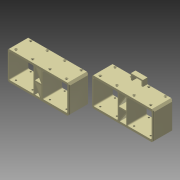
# Autodesk Inventor part: Part6
Saved by Autodesk Inventor 2015 (Build 190159000, 159)
## iProperties
Created: 2015-03-12
Part Number: Part6
Material: Nylon 6/6
Document SubType Name: Modeling
Designer: Vladimir
Density: 1.13 g/cm^3
Appearance: Nylon 6
Author: Vladimir
Autodesk Inventor part; units mm, degrees
ref_plane "YZ Plane" through (0, 0, 0) normal (1, 0, 0) x (0, 1, 0)
ref_plane "XZ Plane" through (0, 0, 0) normal (0, 1, 0) x (-1, 0, 0)
ref_plane "XY Plane" through (0, 0, 0) normal (0, 0, 1) x (1, 0, 0)
sketch "0.2mm tolerance" plane through (0, 0, 0) normal (0, 0, 1) x (1, 0, 0)
  line L0 (-41.2, -0.2479) -> (-41.2, 26.7521)
  line L1 (-13.4, -0.0479) -> (-38, -0.0479)
  line L2 (-39, 0.9521) -> (-39, 25.5521)
  line L3 (-38, 26.5521) -> (-13.4, 26.5521)
  line L4 (-12.4, 25.5521) -> (-12.4, 0.9521)
  line L5 (-1.4, 0.1521) -> (23.2, 0.1521)
  line L6 (24.2, 1.1521) -> (24.2, 25.7521)
  line L7 (23.2, 26.7521) -> (-1.4, 26.7521)
  line L8 (-2.4, 25.7521) -> (-2.4, 1.1521)
  line L9 (26.4, -0.2479) -> (26.4, 26.7521)
  line L10 (-39.2, -2.2479) -> (24.4, -2.2479)
  line L11 (-39.2, 28.7521) -> (24.4, 28.7521)
  line L12 (-10.9, 12.0286) -> (-3.9, -0.0479)
  line L13 (-5.287, -0.0479) -> (-10.9, 9.6357)
  line L14 (-5.287, -0.0479) -> (-10.9, -0.0479)
  line L15 (-3.9, -0.0479) -> (-3.9, 12.0286)
  line L16 (-10.9, 9.6357) -> (-10.9, -0.0479)
  line L17 (-10.9, 12.0286) -> (-3.9, 12.0286)
  arc A0 (-1.4, 26.7521) -> (-2.4, 25.7521) centre (-1.4, 25.7521) ccw
  arc A1 (-2.4, 1.1521) -> (-1.4, 0.1521) centre (-1.4, 1.1521) ccw
  arc A2 (23.2, 0.1521) -> (24.2, 1.1521) centre (23.2, 1.1521) ccw
  arc A3 (24.2, 25.7521) -> (23.2, 26.7521) centre (23.2, 25.7521) ccw
  arc A4 (-38, 26.5521) -> (-39, 25.5521) centre (-38, 25.5521) ccw
  arc A5 (-12.4, 25.5521) -> (-13.4, 26.5521) centre (-13.4, 25.5521) ccw
  arc A6 (-13.4, -0.0479) -> (-12.4, 0.9521) centre (-13.4, 0.9521) ccw
  arc A7 (-39, 0.9521) -> (-38, -0.0479) centre (-38, 0.9521) ccw
  line L18 (24.4, -2.2479) -> (26.4, -0.2479)
  line L19 (24.4, 28.7521) -> (26.4, 26.7521)
  line L20 (-41.2, -0.2479) -> (-39.2, -2.2479)
  line L21 (-39.2, 28.7521) -> (-41.2, 26.7521)
  line L22 (-3.9, 13.5286) -> (-10.9, 26.5521)
  line L23 (-9.5376, 26.5521) -> (-3.9, 16.0632)
  line L24 (-9.5376, 26.5521) -> (-3.9, 26.5521)
  line L25 (-10.9, 26.5521) -> (-10.9, 13.5286)
  line L26 (-3.9, 16.0632) -> (-3.9, 26.5521)
  line L27 (-3.9, 13.5286) -> (-10.9, 13.5286)
  point P0 (0, 0)
  point P1 (-41.2, 28.7521)
  point P2 (-41.2, -2.2479)
  point P3 (-12.4, -0.0479)
  point P4 (-39, 26.5521)
  point P5 (-39, -0.0479)
  point P6 (-12.4, 26.5521)
  point P7 (24.2, 26.7521)
  point P8 (-2.4, 26.7521)
  point P9 (26.4, 28.7521)
  point P10 (26.4, -2.2479)
  dimension "d11" = 31
  dimension "d12" = 26.6
  dimension "d13" = 26.6
  dimension "d14" = 26.6
  dimension "d46" = 2.2
  dimension "d47" = 2.2
  dimension "d48" = 67.6
  dimension "d68" = 1
  dimension "d69" = 1
  dimension "d70" = 1
  dimension "d71" = 1
  dimension "d72" = 1
  dimension "d73" = 1
  dimension "d74" = 1
  dimension "d75" = 1
  dimension "d76" = 2
  dimension "d77" = 2
  dimension "d78" = 2
  dimension "d79" = 2
  dimension "d80" = 2
  dimension "d81" = 2
  dimension "d82" = 2
  dimension "d83" = 2
  dimension "d253" = 26.6
  dimension "d254" = 1.5
  dimension "d255" = 1.2
  dimension "d263" = 2.2
  dimension "d267" = 2.2
  dimension "d268" = 2.2
  dimension "d273" = 1.5
  dimension "d277" = 10
  dimension "d279" = 2.2
  dimension "d280" = 2.2
  dimension "d281" = 2.2
  dimension "d282" = 1.5
  dimension "d283" = 1.2
  dimension "d284" = 1.5
  dimension "d285" = 1.5
  dimension "d286" = 1.5
  dimension "d287" = 1.5
  constraints: 56 end point, 20 point on line, 16 point on circle, 16 tangent, 8 centre point, 6 parallel, 6 perpendicular, 5 horizontal, 1 vertical
  measures "d11" distance of point (-41.2, -2.248) point (-41.2, 28.752)
  measures "d12" distance of point (-39, 26.552) point (-12.4, 26.552)
  measures "d13" distance of point (-39, -0.048) point (-39, 26.552)
  measures "d14" distance of point (-2.4, 26.752) point (24.2, 26.752)
  measures "d46" distance between parallel lines of L9 L6
  measures "d47" distance between parallel lines of L0 L2
  measures "d48" distance of point (-41.2, 28.752) point (26.4, 28.752)
  measures "d68" radius of A0
  measures "d69" radius of A1
  measures "d70" radius of A2
  measures "d71" radius of A3
  measures "d72" radius of A4
  measures "d73" radius of A5
  measures "d74" radius of A6
  measures "d75" radius of A7
  measures "d76" distance of L10.end point (26.4, -2.248)
  measures "d77" distance of L9.start point (26.4, -2.248)
  measures "d78" distance of L11.end point (26.4, 28.752)
  measures "d79" distance of L9.end point (26.4, 28.752)
  measures "d80" distance of L0.start point (-41.2, -2.248)
  measures "d81" distance of L10.start point (-41.2, -2.248)
  measures "d82" distance of L11.start point (-41.2, 28.752)
  measures "d83" distance of L0.end point (-41.2, 28.752)
  measures "d253" distance between parallel lines of L5 L7
  measures "d254" distance between parallel lines of L8 L15
  measures "d255" distance between parallel lines of L12 L13
  measures "d263" distance between parallel lines of L10 L14
  measures "d267" distance between parallel lines of L3 L11
  measures "d268" distance between parallel lines of L10 L1
  measures "d273" distance between parallel lines of L4 L16
  measures "d277" distance between parallel lines of L8 L4
  measures "d279" distance from line of L10 L12.end
  measures "d280" distance from line of L11 L25.start
  measures "d281" distance between parallel lines of L11 L24
  measures "d282" distance between parallel lines of L17 L27
  measures "d283" distance between parallel lines of L23 L22
  measures "d284" distance from line of L4 L12.start
  measures "d285" distance between parallel lines of L4 L25
  measures "d286" distance between parallel lines of L8 L26
  measures "d287" distance from line of L8 L22.start
extrude "Vol 0.2 mm" add sketch "0.2mm tolerance" along normal blind 21
sketch "0.2 mm mounting hole" plane through (-39.2, 28.7521, 0) normal (0, 1, 0) x (1, 0, 0)
  line L0 (-2, 0) -> (65.822, 0)
  line L1 (65.822, 0) -> (65.822, -21)
  line L2 (65.822, -21) -> (-2, -21)
  line L3 (-2, -21) -> (-2, 0)
  line L4 (0, -21) -> (63.6, -21) projected
  line L5 (-2, 0) -> (0.3, 0)
  line L6 (0.3, 0) -> (0.3, -21)
  line L7 (0.3, -21) -> (-2, -21)
  line L8 (-2, -21) -> (-2, 0)
  line L9 (0.3, 0) -> (26.7, 0)
  line L10 (26.7, 0) -> (26.7, -21)
  line L11 (26.7, -21) -> (0.3, -21)
  line L12 (0.3, -21) -> (0.3, 0)
  line L13 (65.822, -21) -> (63.522, -21)
  line L14 (63.522, -21) -> (63.522, 0)
  line L15 (63.522, 0) -> (65.822, 0)
  line L16 (65.822, 0) -> (65.822, -21)
  line L17 (0, 0) -> (63.6, 0) projected
  line L18 (63.522, -21) -> (37.122, -21)
  line L19 (37.122, -21) -> (37.122, 0)
  line L20 (37.122, 0) -> (63.522, 0)
  line L21 (63.522, 0) -> (63.522, -21)
  circle A0 centre (59.322, -1.7) radius 0.95
  circle A1 centre (41.322, -1.7) radius 0.95
  circle A2 centre (59.322, -17.7) radius 0.95
  circle A3 centre (41.322, -17.7) radius 0.95
  circle A4 centre (22.5, -1.7) radius 0.95
  circle A5 centre (4.5, -1.7) radius 0.95
  circle A6 centre (4.5, -17.7) radius 0.95
  circle A7 centre (22.5, -17.7) radius 0.95
  point P0 (39.2, 0)
  dimension "d296" = 2.3
  dimension "d297" = 26.4
  dimension "d298" = 2.3
  dimension "d299" = 26.4
  dimension "d300" = 1.9
  dimension "d301" = 1.9
  dimension "d302" = 18
  dimension "d303" = 4.2
  dimension "d304" = 4.2
  dimension "d305" = 1.7
  dimension "d306" = 1.9
  dimension "d307" = 1.9
  dimension "d308" = 16
  dimension "d309" = 16
  dimension "d310" = 1.9
  dimension "d311" = 1.9
  dimension "d312" = 1.9
  dimension "d313" = 1.9
  dimension "d314" = 16
  dimension "d315" = 1.7
  dimension "d316" = 1.7
  dimension "d317" = 18
  dimension "d318" = 4.2
  dimension "d319" = 4.2
  dimension "d320" = 4.2
  dimension "d321" = 4.2
  dimension "d322" = 16
  dimension "d323" = 18
  constraints: 40 end point, 10 parallel, 8 centre point, 5 horizontal, 5 perpendicular, 4 point on line
  measures "d296" distance of L6.end L7.end
  measures "d297" distance of L10.end L11.end
  measures "d298" distance of L14.end L15.end
  measures "d299" distance of L19.end L20.end
  measures "d300" diameter of A0
  measures "d301" diameter of A1
  measures "d302" distance of A1.centre A0.centre
  measures "d303" distance from line of A0.centre L21
  measures "d304" distance from line of L19 A1.centre
  measures "d305" distance from line of L20 A0.centre
  measures "d306" diameter of A2
  measures "d307" diameter of A3
  measures "d308" distance of A0.centre A2.centre
  measures "d309" distance of A1.centre A3.centre
  measures "d310" diameter of A4
  measures "d311" diameter of A5
  measures "d312" diameter of A6
  measures "d313" diameter of A7
  measures "d314" distance of A7.centre A4.centre
  measures "d315" distance from line of L9 A4.centre
  measures "d316" distance from line of L9 A5.centre
  measures "d317" distance of A4.centre A5.centre
  measures "d318" distance from line of L10 A4.centre
  measures "d319" distance from line of L6 A5.centre
  measures "d320" distance from line of L10 A7.centre
  measures "d321" distance from line of L6 A6.centre
  measures "d322" distance of A5.centre A6.centre
  measures "d323" distance of A6.centre A7.centre
hole "Hole 0.2mm" at (-41.2, 28.7521, 0) at (20.122, 28.7521, 1.7) at (20.122, 28.7521, 17.7) at (2.122, 28.7521, 17.7) at (2.122, 28.7521, 1.7) at (-16.7, 28.7521, 17.7) at (-16.7, 28.7521, 1.7) at (-34.7, 28.7521, 17.7) at (-34.7, 28.7521, 1.7) at (-41.2, 28.7521, 21) at (26.622, 28.7521, 21) at (26.622, 28.7521, 0) direction (0, -1, 0) diameter 1.9 end through all counterbore diameter 3 counterbore depth 0.5
sketch "0.1 tolerance" plane through (-14.365, -0.3025, 0) normal (0, 0, -1) x (-1, 0, 0)
  line L0 (-111.2019, 0.0288) -> (-111.2019, 27.0288)
  line L1 (-83.7019, 0.2788) -> (-107.8019, 0.2788)
  line L2 (-109.0019, 1.4788) -> (-109.0019, 25.5788)
  line L3 (-107.8019, 26.7788) -> (-83.7019, 26.7788)
  line L4 (-82.5019, 25.5788) -> (-82.5019, 1.4788)
  line L5 (-71.1019, 0.2288) -> (-47.0019, 0.2288)
  line L6 (-45.8019, 1.4288) -> (-45.8019, 25.5788)
  line L7 (-47.0019, 26.7788) -> (-71.1019, 26.7788)
  line L8 (-72.3019, 25.5788) -> (-72.3019, 1.4288)
  line L9 (-43.6019, 0.0288) -> (-43.6019, 27.0288)
  line L10 (-109.2019, -1.9712) -> (-45.6019, -1.9712)
  line L11 (-109.2019, 29.0288) -> (-45.6019, 29.0288)
  line L12 (-81.5019, 12.3053) -> (-73.3019, 0.2288)
  line L13 (-74.5107, 0.2288) -> (-81.5019, 10.5251)
  line L14 (-74.5107, 0.2288) -> (-81.5019, 0.2288)
  line L15 (-73.3019, 0.2288) -> (-73.3019, 12.3053)
  line L16 (-81.5019, 10.5251) -> (-81.5019, 0.2288)
  line L17 (-81.5019, 12.3053) -> (-73.3019, 12.3053)
  arc A0 (-71.1019, 26.7788) -> (-72.3019, 25.5788) centre (-71.1019, 25.5788) ccw
  arc A1 (-72.3019, 1.4288) -> (-71.1019, 0.2288) centre (-71.1019, 1.4288) ccw
  arc A2 (-47.0019, 0.2288) -> (-45.8019, 1.4288) centre (-47.0019, 1.4288) ccw
  arc A3 (-45.8019, 25.5788) -> (-47.0019, 26.7788) centre (-47.0019, 25.5788) ccw
  arc A4 (-107.8019, 26.7788) -> (-109.0019, 25.5788) centre (-107.8019, 25.5788) ccw
  arc A5 (-82.5019, 25.5788) -> (-83.7019, 26.7788) centre (-83.7019, 25.5788) ccw
  arc A6 (-83.7019, 0.2788) -> (-82.5019, 1.4788) centre (-83.7019, 1.4788) ccw
  arc A7 (-109.0019, 1.4788) -> (-107.8019, 0.2788) centre (-107.8019, 1.4788) ccw
  line L18 (-45.6019, -1.9712) -> (-43.6019, 0.0288)
  line L19 (-45.6019, 29.0288) -> (-43.6019, 27.0288)
  line L20 (-111.2019, 0.0288) -> (-109.2019, -1.9712)
  line L21 (-109.2019, 29.0288) -> (-111.2019, 27.0288)
  line L22 (-80.3189, 26.7788) -> (-73.3019, 26.7788)
  line L23 (-81.5019, 26.7788) -> (-81.5019, 13.8053)
  line L24 (-80.3189, 26.7788) -> (-73.3019, 15.6769)
  line L25 (-73.3019, 15.6769) -> (-73.3019, 26.7788)
  line L26 (-73.3019, 13.8053) -> (-81.5019, 26.7788)
  line L27 (-73.3019, 13.8053) -> (-81.5019, 13.8053)
  point P0 (-70.0019, 0.2767)
  point P1 (-111.2019, 29.0288)
  point P2 (-111.2019, -1.9712)
  point P3 (-82.5019, 0.2788)
  point P4 (-109.0019, 26.7788)
  point P5 (-109.0019, 0.2788)
  point P6 (-82.5019, 26.7788)
  point P7 (-45.8019, 26.7788)
  point P8 (-72.3019, 26.7788)
  point P9 (-43.6019, 29.0288)
  point P10 (-43.6019, -1.9712)
  dimension "d368" = 31
  dimension "d366" = 26.5
  dimension "d367" = 26.5
  dimension "d364" = 26.5
  dimension "d361" = 2.2
  dimension "d365" = 2.2
  dimension "d362" = 67.6
  dimension "d353" = 1.2
  dimension "d352" = 1.2
  dimension "d351" = 1.2
  dimension "d350" = 1.2
  dimension "d349" = 1.2
  dimension "d348" = 1.2
  dimension "d347" = 1.2
  dimension "d346" = 1.2
  dimension "d345" = 2
  dimension "d344" = 2
  dimension "d343" = 2
  dimension "d342" = 2
  dimension "d341" = 2
  dimension "d340" = 2
  dimension "d339" = 2
  dimension "d338" = 2
  dimension "d363" = 26.55
  dimension "d355" = 1
  dimension "d357" = 1
  dimension "d356" = 2.2
  dimension "d360" = 2.25
  dimension "d372" = 2.25
  dimension "d354" = 1
  dimension "d373" = 10.2
  dimension "d358" = 2.2
  dimension "d337" = 2.25
  dimension "d336" = 2.25
  dimension "d331" = 1.5
  dimension "d333" = 1
  dimension "d359" = 1
  dimension "d335" = 1
  dimension "d334" = 1
  dimension "d332" = 1
  dimension "d410" = 2.25
  constraints: 56 end point, 20 point on line, 16 point on circle, 16 tangent, 8 centre point, 6 parallel, 6 perpendicular, 5 horizontal, 1 vertical
  measures "d368" distance of point (-111.202, -1.971) point (-111.202, 29.029)
  measures "d366" distance of point (-109.002, 26.779) point (-82.502, 26.779)
  measures "d367" distance of point (-109.002, 0.279) point (-109.002, 26.779)
  measures "d364" distance of point (-72.302, 26.779) point (-45.802, 26.779)
  measures "d361" distance between parallel lines of L9 L6
  measures "d365" distance between parallel lines of L0 L2
  measures "d362" distance of point (-111.202, 29.029) point (-43.602, 29.029)
  measures "d353" radius of A0
  measures "d352" radius of A1
  measures "d351" radius of A2
  measures "d350" radius of A3
  measures "d349" radius of A4
  measures "d348" radius of A5
  measures "d347" radius of A6
  measures "d346" radius of A7
  measures "d345" distance of L10.end point (-43.602, -1.971)
  measures "d344" distance of L9.start point (-43.602, -1.971)
  measures "d343" distance of L11.end point (-43.602, 29.029)
  measures "d342" distance of L9.end point (-43.602, 29.029)
  measures "d341" distance of L0.start point (-111.202, -1.971)
  measures "d340" distance of L10.start point (-111.202, -1.971)
  measures "d339" distance of L11.start point (-111.202, 29.029)
  measures "d338" distance of L0.end point (-111.202, 29.029)
  measures "d363" distance between parallel lines of L5 L7
  measures "d355" distance between parallel lines of L8 L15
  measures "d357" distance between parallel lines of L12 L13
  measures "d356" distance between parallel lines of L10 L14
  measures "d360" distance between parallel lines of L3 L11
  measures "d372" distance between parallel lines of L10 L1
  measures "d354" distance between parallel lines of L4 L16
  measures "d373" distance between parallel lines of L8 L4
  measures "d358" distance from line of L10 L12.end
  measures "d337" distance from line of L11 L23.start
  measures "d336" distance between parallel lines of L11 L22
  measures "d331" distance between parallel lines of L17 L27
  measures "d333" distance between parallel lines of L24 L26
  measures "d359" distance from line of L4 L12.start
  measures "d335" distance between parallel lines of L4 L23
  measures "d334" distance between parallel lines of L8 L25
  measures "d332" distance from line of L8 L26.start
  measures "d410" distance between parallel lines of L7 L11
extrude "0.1 mm tolerance" add sketch "0.1 tolerance" along normal blind 21
sketch "Sketch11" plane through (65.037, 28.7262, -10.5) normal (0, 1, 0) x (1, 0, 0)
  line L0 (-35.8, 10.5) -> (31.8, 10.5)
  line L1 (31.8, 10.5) -> (31.8, -10.5)
  line L2 (31.8, -10.5) -> (-35.8, -10.5)
  line L3 (-35.8, -10.5) -> (-35.8, 10.5)
  line L4 (-33.8499, -10.5) -> (29.7501, -10.5)
  line L5 (-35.8, 10.5) -> (-33.55, 10.5)
  line L6 (-33.55, 10.5) -> (-33.55, -10.5)
  line L7 (-33.55, -10.5) -> (-35.8, -10.5)
  line L8 (-35.8, -10.5) -> (-35.8, 10.5)
  line L9 (-33.55, 10.5) -> (-7.15, 10.5)
  line L10 (-7.15, 10.5) -> (-7.15, -10.5)
  line L11 (-7.15, -10.5) -> (-33.55, -10.5)
  line L12 (-33.55, -10.5) -> (-33.55, 10.5)
  line L13 (31.8, -10.5) -> (29.55, -10.5)
  line L14 (29.55, -10.5) -> (29.55, 10.5)
  line L15 (29.55, 10.5) -> (31.8, 10.5)
  line L16 (31.8, 10.5) -> (31.8, -10.5)
  line L17 (-33.9719, 10.5) -> (29.6281, 10.5)
  line L18 (29.55, -10.5) -> (3.15, -10.5)
  line L19 (3.15, -10.5) -> (3.15, 10.5)
  line L20 (3.15, 10.5) -> (29.55, 10.5)
  line L21 (29.55, 10.5) -> (29.55, -10.5)
  circle A0 centre (25.35, 8.8) radius 0.95
  circle A1 centre (7.35, 8.8) radius 0.95
  circle A2 centre (25.3501, -7.2) radius 0.95
  circle A3 centre (7.3501, -7.2) radius 0.95
  circle A4 centre (-11.35, 8.8) radius 0.95
  circle A5 centre (-29.35, 8.8) radius 0.95
  circle A6 centre (-29.35, -7.2) radius 0.95
  circle A7 centre (-11.35, -7.2) radius 0.95
  point P0 (5.2281, 10.5)
  dimension "d400" = 2.25
  dimension "d399" = 26.4
  dimension "d398" = 2.25
  dimension "d397" = 26.4
  dimension "d394" = 1.9
  dimension "d391" = 1.9
  dimension "d393" = 18
  dimension "d396" = 4.2
  dimension "d392" = 4.2
  dimension "d395" = 1.7
  dimension "d389" = 1.9
  dimension "d387" = 1.9
  dimension "d390" = 16
  dimension "d388" = 16
  dimension "d384" = 1.9
  dimension "d381" = 1.9
  dimension "d378" = 1.9
  dimension "d375" = 1.9
  dimension "d377" = 16
  dimension "d386" = 1.7
  dimension "d383" = 1.7
  dimension "d382" = 18
  dimension "d385" = 4.2
  dimension "d407" = 4.2
  dimension "d376" = 4.2
  dimension "d380" = 4.2
  dimension "d379" = 16
  dimension "d408" = 18
  dimension "d409" = 67.6
  constraints: 44 end point, 10 parallel, 8 centre point, 5 horizontal, 5 perpendicular, 4 point on line, 1 vertical
  measures "d400" distance of L6.end L7.end
  measures "d399" distance of L10.end L11.end
  measures "d398" distance of L14.end L15.end
  measures "d397" distance of L19.end L20.end
  measures "d394" diameter of A0
  measures "d391" diameter of A1
  measures "d393" distance of A1.centre A0.centre
  measures "d396" distance from line of A0.centre L21
  measures "d392" distance from line of L19 A1.centre
  measures "d395" distance from line of L20 A0.centre
  measures "d389" diameter of A2
  measures "d387" diameter of A3
  measures "d390" distance of A0.centre A2.centre
  measures "d388" distance of A1.centre A3.centre
  measures "d384" diameter of A4
  measures "d381" diameter of A5
  measures "d378" diameter of A6
  measures "d375" diameter of A7
  measures "d377" distance of A7.centre A4.centre
  measures "d386" distance from line of L9 A4.centre
  measures "d383" distance from line of L9 A5.centre
  measures "d382" distance of A4.centre A5.centre
  measures "d385" distance from line of L10 A4.centre
  measures "d407" distance from line of L6 A5.centre
  measures "d376" distance from line of L10 A7.centre
  measures "d380" distance from line of L6 A6.centre
  measures "d379" distance of A5.centre A6.centre
  measures "d408" distance of A6.centre A7.centre
  measures "d409" distance between parallel lines of L8 L1
hole "Hole7" at (29.237, 28.7262, -21) at (90.387, 28.7262, -19.3) at (90.3871, 28.7262, -3.3) at (72.3871, 28.7262, -3.3) at (72.387, 28.7262, -19.3) at (53.687, 28.7262, -3.3) at (53.687, 28.7262, -19.3) at (35.687, 28.7262, -3.3) at (35.687, 28.7262, -19.3) at (29.237, 28.7262, 0) at (96.837, 28.7262, 0) at (96.837, 28.7262, -21) direction (0, -1, 0) diameter 1.9 end through all counterbore diameter 3 counterbore depth 0.5
sketch "Sketch12" plane through (-14.365, -0.3025, -21) normal (0, 0, -1) x (-1, 0, 0)
  line L0 (-109.2019, -1.9712) -> (-45.6019, -1.9712) projected
  line L1 (-70.3283, -1.9712) -> (-83.3283, -1.9712)
  line L2 (-83.3283, -1.9712) -> (-83.3283, -8.4712)
  line L3 (-83.3283, -8.4712) -> (-70.3283, -8.4712)
  line L4 (-70.3283, -8.4712) -> (-70.3283, -1.9712)
  line L5 (-71.8283, -1.9712) -> (-81.8287, -1.9712)
  line L6 (-81.8287, -1.9712) -> (-81.8287, -6.9712)
  line L7 (-81.8287, -6.9712) -> (-71.8283, -6.9712)
  line L8 (-71.8283, -6.9712) -> (-71.8283, -1.9712)
  line L9 (-83.5036, 28.9683) -> (-70.5036, 28.9683)
  line L10 (-70.5036, 28.9683) -> (-70.5036, 35.4683)
  line L11 (-70.5036, 35.4683) -> (-83.5036, 35.4683)
  line L12 (-83.5036, 35.4683) -> (-83.5036, 28.9683)
  line L13 (-82.0036, 28.9683) -> (-72.0032, 28.9683)
  line L14 (-72.0032, 28.9683) -> (-72.0032, 33.9683)
  line L15 (-72.0032, 33.9683) -> (-82.0036, 33.9683)
  line L16 (-82.0036, 33.9683) -> (-82.0036, 28.9683)
  point P0 (-14.365, 0.3025)
  dimension "d411" = 13
  dimension "d412" = 6.5
  dimension "d413" = 1.4996
  dimension "d414" = 1.5
  dimension "d415" = 1.5
  dimension "d416" = 13
  dimension "d417" = 6.5
  dimension "d418" = 1.4996
  dimension "d419" = 1.5
  dimension "d420" = 1.5
  constraints: 32 end point, 8 parallel, 4 perpendicular, 3 point on line, 2 horizontal
  measures "d411" distance of L3.end L2.end
  measures "d412" distance of L2.end L1.end
  measures "d413" distance between parallel lines of L2 L6
  measures "d414" distance between parallel lines of L4 L8
  measures "d415" distance between parallel lines of L3 L7
  measures "d416" distance of L11.end L10.end
  measures "d417" distance of L10.end L9.end
  measures "d418" distance between parallel lines of L10 L14
  measures "d419" distance between parallel lines of L12 L16
  measures "d420" distance between parallel lines of L11 L15
extrude "Extrusion6" add sketch "Sketch12" against normal blind 5 contours L0 L6 L7 L8 L4 L3 L2 | L12 L11 L10 L9 L14 L15 L16
body "Solid1"
